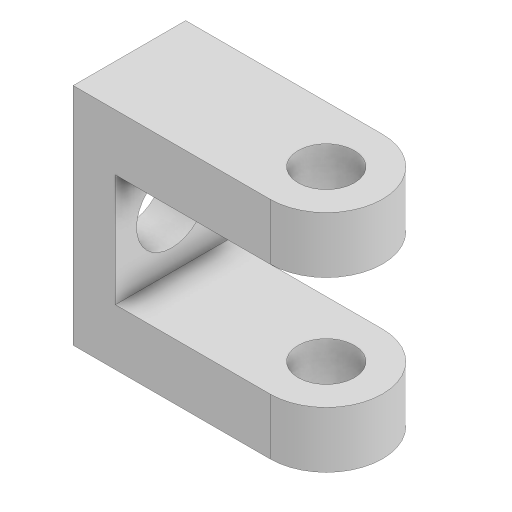
# Autodesk Inventor part: actuator mount 2
Saved by Autodesk Inventor 2023 (Build 270158000, 158)
## iProperties
Created: 2023-07-19
Part Number: actuator mount 2
Material: Generic
Document SubType Name: Modeling
Designer: Juyoung Han
Density: 1 g/cm^3
Appearance: Default
Author: Juyoung Han
Autodesk Inventor part; units mm, degrees
ref_plane "YZ Plane" through (0, 0, 0) normal (1, 0, 0) x (0, 1, 0)
ref_plane "XZ Plane" through (0, 0, 0) normal (0, 1, 0) x (-1, 0, 0)
ref_plane "XY Plane" through (0, 0, 0) normal (0, 0, 1) x (1, 0, 0)
sketch "Sketch1" plane through (0, 0, 0) normal (0, 0, 1) x (1, 0, 0)
  line L0 (0, 0) -> (0, 4)
  line L1 (0, 4) -> (15, 4)
  line L2 (15, 4) -> (15, 8)
  line L3 (15, 8) -> (-3, 8)
  line L4 (-3, 8) -> (-3, 0)
  line L5 (0, 0) -> (0, -4)
  line L6 (0, -4) -> (15, -4)
  line L7 (15, -4) -> (15, -8)
  line L8 (15, -8) -> (-3, -8)
  line L9 (-3, -8) -> (-3, 0)
  point P0 (0, 2)
  dimension "d4" = 3
  dimension "d5" = 4
  dimension "d17" = 15
  constraints: 20 end point, 4 perpendicular, 1 midpoint, 1 vertical
  measures "d4" distance from line of point (0, 2) L4
  measures "d5" distance between parallel lines of L3 L1
  measures "d17" distance between parallel lines of L7 L5
extrude "Extrusion1" add sketch "Sketch1" along normal blind 8
sketch "Sketch2" plane through (-3, 8, 0) normal (0, 1, 0) x (1, 0, 0)
  circle A0 centre (14, -4) radius 2
  line L0 (18, 0) -> (18, -8) projected
  point P0 (3, 0)
  point P1 (18, -4)
  dimension "d8" = 4
  dimension "d9" = 4
  constraints: 1 centre point, 1 midpoint
  measures "d8" diameter of A0
  measures "d9" distance of A0.centre point (18, -4)
extrude "Extrusion2" cut sketch "Sketch2" against normal through all
fillet "Fillet1" radius 4 4 edges at (15, 6, 8) (15, 6, 0) (15, -6, 8) (15, -6, 0)
sketch "Sketch3" plane through (0, -4, 0) normal (1, 0, 0) x (0, 0, -1)
  circle A0 centre (-4, 4) radius 2.5
  line L0 (0, 0) -> (0, 8) projected
  point P0 (0, 4)
  point P1 (0, 4)
  dimension "d13" = 5
  dimension "d14" = 4
  constraints: 1 centre point, 1 midpoint
  measures "d13" diameter of A0
  measures "d14" distance of point (0, 4) A0.centre
extrude "Extrusion3" cut sketch "Sketch3" against normal blind 10
body "Solid1"
